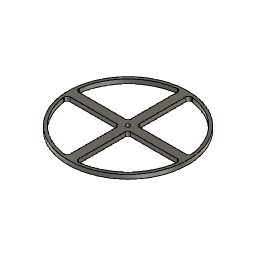
spinning_part_86mm_diameter v2 (Autodesk Fusion 360 design; units mm, degrees)
Autodesk Fusion 360 part; units mm, degrees
sketch "Sketch1" plane through (0, 0, 0) normal (0, 0, 1) x (1, 0, 0)
  circle A0 centre (0, 0) radius 43
  line L0 (-3, 5) -> (-3, 38.6919)
  line L1 (-3, 42.9158) -> (3, 42.9158)
  line L2 (3, 38.6608) -> (3, 5)
  line L3 (5, -3) -> (38.6722, -3)
  line L4 (42.8866, -3) -> (42.8866, 3)
  line L5 (38.7134, 3) -> (5, 3)
  line L6 (3, -5) -> (3, -38.6755)
  line L7 (3, -42) -> (-3, -42)
  line L8 (-3, -38.6545) -> (-3, -5)
  line L9 (-5, 3) -> (-38.6589, 3)
  line L10 (-42.9177, 3) -> (-42.9177, -3)
  line L11 (-38.6701, -3) -> (-5, -3)
  arc A1 (3, 5) -> (5, 3) centre (5, 5) ccw
  arc A2 (5, -3) -> (3, -5) centre (5, -5) ccw
  arc A3 (-3, -5) -> (-5, -3) centre (-5, -5) ccw
  arc A4 (-5, 3) -> (-3, 5) centre (-5, 5) ccw
  line L12 (5.2163, 40.649) -> (5.8611, 40.5789)
  arc A5 (5.2163, 40.649) -> (3, 38.6608) centre (5, 38.6608) ccw
  line L13 (-5.1884, 40.683) -> (-4.7244, 40.7269)
  arc A6 (-3, 38.6919) -> (-5.1884, 40.683) centre (-5, 38.6919) ccw
  arc A7 (38.7134, 3) -> (40.7062, 5.169) centre (38.7134, 5) ccw
  line L14 (40.6615, -5.2061) -> (40.6365, -5.4474)
  arc A8 (40.6615, -5.2061) -> (38.6722, -3) centre (38.6722, -5) ccw
  line L15 (5.2032, -40.6651) -> (5.3266, -40.6525)
  arc A9 (3, -38.6755) -> (5.2032, -40.6651) centre (5, -38.6755) ccw
  line L16 (-5.2218, -40.6421) -> (-6.0887, -40.5454)
  arc A10 (-5.2218, -40.6421) -> (-3, -38.6545) centre (-5, -38.6545) ccw
  line L17 (-40.6592, -5.208) -> (-40.6262, -5.5237)
  arc A11 (-38.6701, -3) -> (-40.6592, -5.208) centre (-38.6701, -5) ccw
  line L18 (-40.647, 5.2179) -> (-40.5692, 5.9278)
  arc A12 (-40.647, 5.2179) -> (-38.6589, 3) centre (-38.6589, 5) ccw
  arc A13 (5.3266, -40.6525) -> (40.6365, -5.4474) centre (0, 0) ccw
  arc A14 (-40.6262, -5.5237) -> (-6.0887, -40.5454) centre (0, 0) ccw
  arc A15 (40.7093, 4.8734) -> (5.8611, 40.5789) centre (0, 0) ccw
  arc A16 (-4.7244, 40.7269) -> (-40.5692, 5.9278) centre (0, 0) ccw
  circle A17 centre (0, 0) radius 1.5
  dimension "d1" = 86
  dimension "d2" = 82
  dimension "d7" = 2
  dimension "d8" = 2
  dimension "d9" = 2
  dimension "d10" = 2
  dimension "d11" = 2
  dimension "d12" = 2
  dimension "d13" = 2
  dimension "d14" = 2
  dimension "d15" = 2
  dimension "d16" = 2
  dimension "d17" = 2
  dimension "d18" = 2
  dimension "d19" = 3
  constraint concentric A0 A15
  constraint vertical L0
  constraint horizontal L1
  constraint vertical L2
  constraint horizontal L3
  constraint vertical L4
  constraint horizontal L5
  constraint vertical L6
  constraint horizontal L7
  constraint vertical L8
  constraint horizontal L9
  constraint vertical L10
  constraint horizontal L11
  constraint tangent L2 A1
  constraint tangent L5 A1
  constraint tangent L6 A2
  constraint tangent L3 A2
  constraint tangent L11 A3
  constraint tangent L8 A3
  constraint tangent L9 A4
  constraint tangent L0 A4
  constraint coincident L1.end L2
  constraint tangent L12 A5
  constraint tangent L2 A5
  constraint coincident L13.end A15
  constraint coincident L1.start L0
  constraint tangent L13 A6
  constraint tangent L0 A6
  constraint coincident L4.end L5
  constraint tangent L5 A7
  constraint coincident L4.start L3
  constraint tangent L3 A8
  constraint tangent L14 A8
  constraint coincident L15.end A15
  constraint coincident L7.start L6
  constraint tangent L15 A9
  constraint tangent L6 A9
  constraint coincident L7.end L8
  constraint tangent L16 A10
  constraint tangent L8 A10
  constraint coincident L17.end A15
  constraint coincident L10.end L11
  constraint tangent L17 A11
  constraint tangent L11 A11
  constraint coincident L10.start L9
  constraint tangent L18 A12
  constraint tangent L9 A12
  constraint coincident A7 A15.start
  constraint concentric A13 A15
  constraint concentric A14 A15
  constraint concentric A15 A16
  constraint concentric A15 A17
  measures "d1" diameter of A0
  measures "d2" diameter of A15
  measures "d7" radius of A1
  measures "d8" radius of A2
  measures "d9" radius of A3
  measures "d10" radius of A4
  measures "d11" radius of A5
  measures "d12" radius of A6
  measures "d13" radius of A7
  measures "d14" radius of A8
  measures "d15" radius of A9
  measures "d16" radius of A10
  measures "d17" radius of A11
  measures "d18" radius of A12
  measures "d19" diameter of A17
extrude "Extrude1" add sketch "Sketch1" along normal blind 3 contours A0 L1 L10
